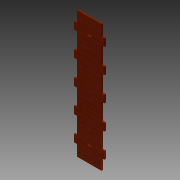
# Autodesk Inventor part: Panel4
Saved by Autodesk Inventor 2015 (Build 190159000, 159)
## iProperties
Created: 2014-08-06
Part Number: Panel4
Material: Wood (Oak)
Document SubType Name: Modeling
Designer: Patrick Camilleri
Density: 0.76 g/cm^3
Appearance: White Oak - Natural Medium Gloss
Author: Patrick Camilleri
Autodesk Inventor part; units mm, degrees
ref_plane "YZ Plane" through (0, 0, 0) normal (1, 0, 0) x (0, 1, 0)
ref_plane "XZ Plane" through (0, 0, 0) normal (0, 1, 0) x (-1, 0, 0)
ref_plane "XY Plane" through (0, 0, 0) normal (0, 0, 1) x (1, 0, 0)
sketch "Sketch1" plane through (0, 0, 0) normal (0, 1, 0) x (-1, 0, 0)
  line L0 (25, 130) -> (-25, 130)
  line L1 (-25, 130) -> (-25, -130)
  line L2 (-25, -130) -> (25, -130)
  line L3 (25, -130) -> (25, 130)
  line L4 (25, 130) -> (-25, -130) construction
  line L5 (-25, 130) -> (25, -130) construction
  line L6 (28, 133) -> (-28, 133) construction
  line L7 (-28, 133) -> (-28, -133) construction
  line L8 (-28, -133) -> (28, -133) construction
  line L9 (28, -133) -> (28, 133) construction
  line L10 (31, 7.5) -> (25, 7.5)
  line L11 (25, 7.5) -> (25, -7.5)
  line L12 (25, -7.5) -> (31, -7.5)
  line L13 (31, -7.5) -> (31, 7.5)
  line L14 (31, 7.5) -> (25, -7.5) construction
  line L15 (25, 7.5) -> (31, -7.5) construction
  line L16 (31, 57.5) -> (25, 57.5)
  line L17 (25, 57.5) -> (25, 42.5)
  line L18 (25, 42.5) -> (31, 42.5)
  line L19 (31, 42.5) -> (31, 57.5)
  line L20 (31, 107.5) -> (25, 107.5)
  line L21 (25, 107.5) -> (25, 92.5)
  line L22 (25, 92.5) -> (31, 92.5)
  line L23 (31, 92.5) -> (31, 107.5)
  line L24 (31, -42.5) -> (25, -42.5)
  line L25 (25, -42.5) -> (25, -57.5)
  line L26 (25, -57.5) -> (31, -57.5)
  line L27 (31, -57.5) -> (31, -42.5)
  line L28 (31, -92.5) -> (25, -92.5)
  line L29 (25, -92.5) -> (25, -107.5)
  line L30 (25, -107.5) -> (31, -107.5)
  line L31 (31, -107.5) -> (31, -92.5)
  line L32 (-25, 7.5) -> (-31, 7.5)
  line L33 (-31, 7.5) -> (-31, -7.5)
  line L34 (-31, -7.5) -> (-25, -7.5)
  line L35 (-25, -7.5) -> (-25, 7.5)
  line L36 (-25, 7.5) -> (-31, -7.5) construction
  line L37 (-31, 7.5) -> (-25, -7.5) construction
  line L38 (-25, -42.5) -> (-31, -42.5)
  line L39 (-31, -42.5) -> (-31, -57.5)
  line L40 (-31, -57.5) -> (-25, -57.5)
  line L41 (-25, -57.5) -> (-25, -42.5)
  line L42 (-25, -92.5) -> (-31, -92.5)
  line L43 (-31, -92.5) -> (-31, -107.5)
  line L44 (-31, -107.5) -> (-25, -107.5)
  line L45 (-25, -107.5) -> (-25, -92.5)
  line L46 (-25, 57.5) -> (-31, 57.5)
  line L47 (-31, 57.5) -> (-31, 42.5)
  line L48 (-31, 42.5) -> (-25, 42.5)
  line L49 (-25, 42.5) -> (-25, 57.5)
  line L50 (-25, 107.5) -> (-31, 107.5)
  line L51 (-31, 107.5) -> (-31, 92.5)
  line L52 (-31, 92.5) -> (-25, 92.5)
  line L53 (-25, 92.5) -> (-25, 107.5)
  point P0 (0, 0)
  point P1 (28, 0)
  point P2 (-28, 0)
  point P3 (0, 0)
  dimension "d0" = 50
  dimension "d1" = 260
  dimension "d2" = 3
  dimension "d3" = 15
  dimension "d6" = 50
  dimension "d13" = 50
  dimension "d18" = 6
  dimension "d19" = 15
  dimension "d22" = 50
  dimension "d29" = 50
  constraints: 108 end point, 9 midpoint, 8 parallel, 4 perpendicular, 4 vertical, 3 horizontal, 1 point on line, 67 other
  measures "d0" distance of L2.end L1.end
  measures "d1" distance of L1.end L0.end
  measures "d2" distance between parallel lines of L3 L9
  measures "d3" distance of L11.end L10.end
  measures "d6" distance of L10.start L16.start
  measures "d13" distance of L12.end L27.start
  measures "d18" distance of L34.end L33.end
  measures "d19" distance of L33.end L32.end
  measures "d22" distance of L34.end L41.start
  measures "d29" distance of L34.end L49.start
extrude "Extrusion1" add sketch "Sketch1" along normal blind 3
sketch "Sketch2" plane through (0, 0, 0) normal (0, -1, 0) x (1, 0, 0)
  line L0 (-4.15, -96) -> (4.15, -96)
  line L1 (4.15, -96) -> (4.15, -99)
  line L2 (4.15, -99) -> (-4.15, -99)
  line L3 (-4.15, -99) -> (-4.15, -96)
  line L4 (-4.15, -96) -> (4.15, -99) construction
  line L5 (4.15, -96) -> (-4.15, -99) construction
  line L6 (-44.7275, 0) -> (39.9331, 0) construction
  line L7 (-4.15, 96) -> (4.15, 96)
  line L8 (4.15, 96) -> (4.15, 99)
  line L9 (4.15, 99) -> (-4.15, 99)
  line L10 (-4.15, 99) -> (-4.15, 96)
  point P0 (0, 0)
  point P1 (0, -97.5)
  dimension "d41" = 8.3
  dimension "d42" = 3
  dimension "d46" = 96
  constraints: 22 end point, 4 symmetric about line, 2 horizontal, 2 midpoint, 2 parallel, 1 perpendicular
  measures "d41" distance of L1.end L2.end
  measures "d42" distance of L0.end L1.end
  measures "d46" distance from line of point (0, 0) L0
extrude "Extrusion2" cut sketch "Sketch2" against normal blind 3
body "Solid1"
